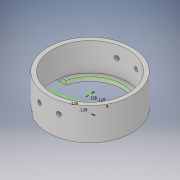
# Autodesk Inventor part: loader20190318_part2
Saved by Autodesk Inventor 2018 (Build 220112000, 112)
## iProperties
Created: 2018-12-11
Part Number: loader20190318_part2
Material: Generic
Document SubType Name: Modeling
Designer: Kim
Density: 1 g/cm^3
Appearance: Default
Author: Kim
Autodesk Inventor part; units mm, degrees
ref_plane "YZ Plane" through (0, 0, 0) normal (1, 0, 0) x (0, 1, 0)
ref_plane "XZ Plane" through (0, 0, 0) normal (0, 1, 0) x (-1, 0, 0)
ref_plane "XY Plane" through (0, 0, 0) normal (0, 0, 1) x (1, 0, 0)
sketch "Sketch1" plane through (0, 0, 0) normal (0, 1, 0) x (-1, 0, 0)
  circle A0 centre (0, 0) radius 58.5076
  circle A1 centre (0, 0) radius 64.8576
  dimension "d0" = 117.0153
  dimension "d1" = 129.7153
  constraints: 2 centre point, 2 coincident
  measures "d0" diameter of A0
  measures "d1" diameter of A1
extrude "Extrusion1" add sketch "Sketch1" along normal blind 43.4975
sketch "Sketch2" plane through (0, 0, 0) normal (0, 1, 0) x (-1, 0, 0)
  circle A0 centre (0, 0) radius 51.562
  circle A1 centre (0, 0) radius 64.8576
  dimension "d4" = 103.124
  dimension "d5" = 129.7153
  constraints: 2 centre point, 2 coincident
  measures "d4" diameter of A0
  measures "d5" diameter of A1
extrude "Extrusion2" add sketch "Sketch2" against normal blind 6.35
sketch "Sketch3" plane through (0, 0, 0) normal (0, 1, 0) x (-1, 0, 0)
  circle A0 centre (12.7, 12.7) radius 1.6256
  circle A1 centre (12.7, -12.7) radius 1.6256
  circle A2 centre (-12.7, 12.7) radius 1.6256
  circle A3 centre (-12.7, -12.7) radius 1.6256
  circle A4 centre (0, 0) radius 50.1447
  line L0 (53.4401, 17.2954) -> (47.8331, 15.0494)
  line L1 (0, 0) -> (53.4401, 17.2954)
  line L2 (43.7038, 24.586) -> (45.7401, 24.9855)
  line L3 (53.4401, 17.2954) -> (45.7401, 24.9855)
  line L4 (45.7401, 24.9855) -> (0, 0)
  dimension "d8" = 3.2512
  dimension "d9" = 3.2512
  dimension "d10" = 3.2512
  dimension "d11" = 3.2512
  constraints: 10 end point, 5 centre point, 1 coincident
  measures "d8" diameter of A0
  measures "d9" diameter of A1
  measures "d10" diameter of A2
  measures "d11" diameter of A3
sketch "Sketch5" plane through (0, 0, 0) normal (0, 1, 0) x (-1, 0, 0)
  circle A0 centre (0, 0) radius 64.8576 projected
  arc A1 (64.8576, 0) -> (44.4312, 47.2481) centre (0, 0) ccw
  arc A2 (50.9046, 0) -> (35.0064, 36.9572) centre (0, 0) ccw
  line L0 (35.0064, 36.9572) -> (44.4312, 47.2481)
  line L1 (50.9046, 0) -> (64.8576, 0)
  arc A3 (64.8576, 0) -> (44.4312, 47.2481) centre (0, 0) ccw
  constraints: 8 point on circle, 4 end point, 3 centre point, 3 coincident, 1 horizontal
extrude "Extrusion3" cut sketch "Sketch5" against normal blind 7.62 contours L1 A2 L0 A0 picked at (59.6957, 6.2583)
sketch "Sketch10" plane through (0, 0, 0) normal (0, 0, 1) x (1, 0, 0)
  circle A0 centre (-15.0012, 25.7302) radius 3.2499
  point P0 (0, 0)
  dimension "d27" = 6.4999
  constraints: 1 centre point
  measures "d27" diameter of A0
extrude "Extrusion8" cut sketch "Sketch10" along normal mid plane 152.4
sketch "Sketch11" plane through (0, 0, 0) normal (0, 0, 1) x (1, 0, 0)
  circle A0 centre (15.0012, 25.7302) radius 3.2499
  point P0 (0, 0)
  dimension "d30" = 6.4999
  constraints: 1 centre point
  measures "d30" diameter of A0
extrude "Extrusion9" cut sketch "Sketch11" along normal mid plane 152.4
sketch "Sketch12" plane through (0, -6.35, 0) normal (0, -1, 0) x (1, 0, 0)
  line L0 (-58.5076, 0) -> (-64.8576, 0) projected
  line L1 (-64.8576, 0) -> (-49.4674, 0)
  line L2 (-49.4674, 0) -> (-49.4674, -12.7)
  line L3 (-49.4674, -12.7) -> (-64.8576, -12.7)
  line L4 (-64.8576, -12.7) -> (-64.8576, 0)
  point P0 (0, 0)
  dimension "d33" = 12.7
  constraints: 8 end point, 2 parallel, 1 horizontal, 1 perpendicular
  measures "d33" distance of L1.end L2.end
extrude "Extrusion10" cut sketch "Sketch12" against normal blind 6.35
sketch "Sketch13" plane through (0, -6.35, 0) normal (0, -1, 0) x (1, 0, 0)
  point P0 (0, 0)
sketch "Sketch14" plane through (0, -6.35, 0) normal (0, -1, 0) x (1, 0, 0)
  line L0 (-35.1204, 55.8851) -> (-25.6536, 41.7778)
  line L1 (-25.6536, 41.7778) -> (-33.019, 34.9455)
  line L2 (-44.4312, 47.2481) -> (-40.1421, 42.5648) projected
  line L3 (-44.4312, 47.2481) -> (-48.028, 43.8657)
  circle A0 centre (0, 0) radius 64.8576 projected
  line L4 (-48.028, 43.8657) -> (-35.1204, 32.9693)
  line L5 (-35.1204, 32.9693) -> (-33.019, 34.9455)
  line L6 (-48.028, 43.8657) -> (-45.6028, 48.5109)
  line L7 (-45.6028, 48.5109) -> (-35.1204, 55.8851)
  dimension "d36" = 12.7
  constraints: 14 end point, 1 parallel, 2 other
  measures "d36" distance of L2.start L0.start
extrude "Extrusion11" cut sketch "Sketch14" against normal blind 6.35 contours L0 A0 L3 L6 L7 | L0 L1 L5 L4 A0 | A0 L4 L3 picked at (-33.3184, 42.2486)
body "Solid1"
